Autodesk Fusion 360 part; units mm, degrees
(part 2 of 4)
  spline S104 degree 3 poles (141.5126, -71.1186) (141.7888, -71.118) (142.0126, -70.8942) (142.0127, -70.6185) knots 0 0 0 0 1 1 1 1
  line L150 (142.0127, -70.6185) -> (142.0127, -57.6177)
  spline S105 degree 3 poles (142.0127, -57.6177) (142.0126, -57.342) (141.7888, -57.1181) (141.5126, -57.1177) knots 0 0 0 0 1 1 1 1
  line L151 (141.5126, -57.1177) -> (137.5127, -57.1172)
  line L152 (137.5127, -57.1172) -> (137.5127, -56.6175)
  spline S106 degree 3 poles (137.5127, -56.6175) (137.5126, -56.3418) (137.2888, -56.118) (137.0126, -56.1175) knots 0 0 0 0 1 1 1 1
  line L153 (137.0126, -56.1175) -> (133.0126, -56.1175)
  spline S107 degree 3 poles (133.0126, -56.1175) (132.7365, -56.118) (132.5126, -56.3418) (132.5126, -56.6175) knots 0 0 0 0 1 1 1 1
  line L154 (132.5126, -56.6175) -> (132.5126, -57.1172)
  line L155 (132.5126, -57.1172) -> (128.5126, -57.1177)
  spline S108 degree 3 poles (128.5126, -57.1177) (128.2365, -57.118) (128.0126, -57.342) (128.0126, -57.6177) knots 0 0 0 0 1 1 1 1
  line L156 (128.0126, -57.6177) -> (128.0126, -70.6185)
  spline S109 degree 3 poles (128.0126, -70.6185) (128.0126, -70.8942) (128.2365, -71.1181) (128.5126, -71.1186) knots 0 0 0 0 1 1 1 1
  line L157 (128.5126, -71.1186) -> (132.5126, -71.1191)
  line L158 (132.5126, -71.1191) -> (132.5126, -71.6187)
  spline S110 degree 3 poles (132.5126, -71.6187) (132.5126, -71.8943) (132.7365, -72.1181) (133.0126, -72.1187) knots 0 0 0 0 1 1 1 1
  line L159 (133.0126, -72.1187) -> (137.0126, -72.1187)
  spline S111 degree 3 poles (137.0126, -72.1187) (137.2888, -72.1182) (137.5126, -71.8943) (137.5127, -71.6187) knots 0 0 0 0 1 1 1 1
  spline S112 degree 3 poles (17.9501, -64.9749) (18.2263, -64.9744) (18.4501, -64.7505) (18.4501, -64.4749) knots 0 0 0 0 1 1 1 1
  line L160 (18.4501, -64.4749) -> (18.4501, -63.9754)
  line L161 (18.4501, -63.9754) -> (22.4501, -63.9748)
  spline S113 degree 3 poles (22.4501, -63.9748) (22.7263, -63.9743) (22.9501, -63.7505) (22.9501, -63.4748) knots 0 0 0 0 1 1 1 1
  line L162 (22.9501, -63.4748) -> (22.9501, -50.474)
  spline S114 degree 3 poles (22.9501, -50.474) (22.9501, -50.1982) (22.7263, -49.9743) (22.4501, -49.9739) knots 0 0 0 0 1 1 1 1
  line L163 (22.4501, -49.9739) -> (18.4501, -49.9736)
  line L164 (18.4501, -49.9736) -> (18.4501, -49.474)
  spline S115 degree 3 poles (18.4501, -49.474) (18.4501, -49.1983) (18.2263, -48.9744) (17.9501, -48.9739) knots 0 0 0 0 1 1 1 1
  line L165 (17.9501, -48.9739) -> (13.9501, -48.9739)
  spline S116 degree 3 poles (13.9501, -48.9739) (13.674, -48.9745) (13.4501, -49.1983) (13.4501, -49.474) knots 0 0 0 0 1 1 1 1
  line L166 (13.4501, -49.474) -> (13.4501, -49.9736)
  line L167 (13.4501, -49.9736) -> (9.4501, -49.9739)
  spline S117 degree 3 poles (9.4501, -49.9739) (9.174, -49.9741) (8.9501, -50.1981) (8.9501, -50.4739) knots 0 0 0 0 1 1 1 1
  line L168 (8.9501, -50.4739) -> (8.9501, -63.4747)
  spline S118 degree 3 poles (8.9501, -63.4747) (8.9501, -63.7504) (9.174, -63.9743) (9.4501, -63.9747) knots 0 0 0 0 1 1 1 1
  line L169 (9.4501, -63.9747) -> (13.4501, -63.9753)
  line L170 (13.4501, -63.9753) -> (13.4501, -64.4748)
  spline S119 degree 3 poles (13.4501, -64.4748) (13.4501, -64.7505) (13.674, -64.9743) (13.9501, -64.9749) knots 0 0 0 0 1 1 1 1
  line L171 (13.9501, -64.9749) -> (17.9501, -64.9749)
  line L172 (42.2626, -64.4749) -> (42.2627, -63.9754)
  line L173 (42.2627, -63.9754) -> (46.2626, -63.9748)
  spline S120 degree 3 poles (46.2626, -63.9748) (46.5388, -63.9743) (46.7626, -63.7505) (46.7627, -63.4748) knots 0 0 0 0 1 1 1 1
  line L174 (46.7627, -63.4748) -> (46.7627, -50.474)
  spline S121 degree 3 poles (46.7627, -50.474) (46.7626, -50.1982) (46.5388, -49.9743) (46.2626, -49.9739) knots 0 0 0 0 1 1 1 1
  line L175 (46.2626, -49.9739) -> (42.2627, -49.9734)
  line L176 (42.2627, -49.9734) -> (42.2626, -49.4738)
  spline S122 degree 3 poles (42.2626, -49.4738) (42.2626, -49.1981) (42.0388, -48.9742) (41.7626, -48.9738) knots 0 0 0 0 1 1 1 1
  line L177 (41.7626, -48.9738) -> (37.7626, -48.9738)
  spline S123 degree 3 poles (37.7626, -48.9738) (37.4865, -48.9743) (37.2626, -49.1981) (37.2626, -49.4738) knots 0 0 0 0 1 1 1 1
  line L178 (37.2626, -49.4738) -> (37.2626, -49.9734)
  line L179 (37.2626, -49.9734) -> (33.2626, -49.9739)
  spline S124 degree 3 poles (33.2626, -49.9739) (32.9865, -49.9742) (32.7626, -50.1982) (32.7626, -50.474) knots 0 0 0 0 1 1 1 1
  line L180 (32.7626, -50.474) -> (32.7626, -63.4748)
  spline S125 degree 3 poles (32.7626, -63.4748) (32.7626, -63.7505) (32.9865, -63.9743) (33.2626, -63.9748) knots 0 0 0 0 1 1 1 1
  line L181 (33.2626, -63.9748) -> (37.2626, -63.9754)
  line L182 (37.2626, -63.9754) -> (37.2626, -64.4749)
  spline S126 degree 3 poles (37.2626, -64.4749) (37.2626, -64.7505) (37.4865, -64.9744) (37.7626, -64.9749) knots 0 0 0 0 1 1 1 1
  line L183 (37.7626, -64.9749) -> (41.7626, -64.9749)
  spline S127 degree 3 poles (41.7626, -64.9749) (42.0388, -64.9744) (42.2626, -64.7505) (42.2626, -64.4749) knots 0 0 0 0 1 1 1 1
  line L184 (61.3126, -59.7124) -> (61.3127, -59.2129)
  line L185 (61.3127, -59.2129) -> (65.3126, -59.2123)
  spline S128 degree 3 poles (65.3126, -59.2123) (65.5888, -59.2118) (65.8126, -58.988) (65.8127, -58.7123) knots 0 0 0 0 1 1 1 1
  line L186 (65.8127, -58.7123) -> (65.8127, -45.7115)
  spline S129 degree 3 poles (65.8127, -45.7115) (65.8126, -45.4357) (65.5888, -45.2118) (65.3126, -45.2114) knots 0 0 0 0 1 1 1 1
  line L187 (65.3126, -45.2114) -> (61.3127, -45.2109)
  line L188 (61.3127, -45.2109) -> (61.3126, -44.7113)
  spline S130 degree 3 poles (61.3126, -44.7113) (61.3126, -44.4356) (61.0888, -44.2117) (60.8126, -44.2113) knots 0 0 0 0 1 1 1 1
  line L189 (60.8126, -44.2113) -> (56.8126, -44.2113)
  spline S131 degree 3 poles (56.8126, -44.2113) (56.5365, -44.2118) (56.3126, -44.4356) (56.3126, -44.7113) knots 0 0 0 0 1 1 1 1
  line L190 (56.3126, -44.7113) -> (56.3126, -45.2109)
  line L191 (56.3126, -45.2109) -> (52.3126, -45.2114)
  spline S132 degree 3 poles (52.3126, -45.2114) (52.0365, -45.2117) (51.8126, -45.4357) (51.8126, -45.7115) knots 0 0 0 0 1 1 1 1
  line L192 (51.8126, -45.7115) -> (51.8126, -58.7123)
  spline S133 degree 3 poles (51.8126, -58.7123) (51.8126, -58.988) (52.0365, -59.2118) (52.3126, -59.2123) knots 0 0 0 0 1 1 1 1
  line L193 (52.3126, -59.2123) -> (56.3126, -59.2129)
  line L194 (56.3126, -59.2129) -> (56.3126, -59.7124)
  spline S134 degree 3 poles (56.3126, -59.7124) (56.3126, -59.988) (56.5365, -60.2119) (56.8126, -60.2124) knots 0 0 0 0 1 1 1 1
  line L195 (56.8126, -60.2124) -> (60.8126, -60.2124)
  spline S135 degree 3 poles (60.8126, -60.2124) (61.0888, -60.2119) (61.3126, -59.988) (61.3126, -59.7124) knots 0 0 0 0 1 1 1 1
  line L196 (80.3626, -57.3312) -> (80.3627, -56.8316)
  line L197 (80.3627, -56.8316) -> (84.3626, -56.8311)
  spline S136 degree 3 poles (84.3626, -56.8311) (84.6388, -56.8305) (84.8626, -56.6067) (84.8627, -56.331) knots 0 0 0 0 1 1 1 1
  line L198 (84.8627, -56.331) -> (84.8627, -43.3302)
  spline S137 degree 3 poles (84.8627, -43.3302) (84.8626, -43.0545) (84.6388, -42.8306) (84.3626, -42.8302) knots 0 0 0 0 1 1 1 1
  line L199 (84.3626, -42.8302) -> (80.3627, -42.8297)
  line L200 (80.3627, -42.8297) -> (80.3626, -42.33)
  spline S138 degree 3 poles (80.3626, -42.33) (80.3626, -42.0543) (80.1388, -41.8305) (79.8626, -41.83) knots 0 0 0 0 1 1 1 1
  line L201 (79.8626, -41.83) -> (75.8626, -41.83)
  spline S139 degree 3 poles (75.8626, -41.83) (75.5865, -41.8305) (75.3626, -42.0543) (75.3626, -42.33) knots 0 0 0 0 1 1 1 1
  line L202 (75.3626, -42.33) -> (75.3626, -42.8297)
  line L203 (75.3626, -42.8297) -> (71.3626, -42.8302)
  spline S140 degree 3 poles (71.3626, -42.8302) (71.0865, -42.8305) (70.8626, -43.0545) (70.8626, -43.3302) knots 0 0 0 0 1 1 1 1
  line L204 (70.8626, -43.3302) -> (70.8626, -56.331)
  spline S141 degree 3 poles (70.8626, -56.331) (70.8626, -56.6067) (71.0865, -56.8306) (71.3626, -56.8311) knots 0 0 0 0 1 1 1 1
  line L205 (71.3626, -56.8311) -> (75.3626, -56.8316)
  line L206 (75.3626, -56.8316) -> (75.3626, -57.3312)
  spline S142 degree 3 poles (75.3626, -57.3312) (75.3626, -57.6068) (75.5865, -57.8306) (75.8626, -57.8312) knots 0 0 0 0 1 1 1 1
  line L207 (75.8626, -57.8312) -> (79.8626, -57.8312)
  spline S143 degree 3 poles (79.8626, -57.8312) (80.1388, -57.8307) (80.3626, -57.6068) (80.3626, -57.3312) knots 0 0 0 0 1 1 1 1
  line L208 (99.4126, -59.7124) -> (99.4127, -59.2129)
  line L209 (99.4127, -59.2129) -> (103.4126, -59.2123)
  spline S144 degree 3 poles (103.4126, -59.2123) (103.6888, -59.2118) (103.9126, -58.988) (103.9127, -58.7123) knots 0 0 0 0 1 1 1 1
  line L210 (103.9127, -58.7123) -> (103.9127, -45.7115)
  spline S145 degree 3 poles (103.9127, -45.7115) (103.9126, -45.4357) (103.6888, -45.2118) (103.4126, -45.2114) knots 0 0 0 0 1 1 1 1
  line L211 (103.4126, -45.2114) -> (99.4127, -45.2109)
  line L212 (99.4127, -45.2109) -> (99.4126, -44.7113)
  spline S146 degree 3 poles (99.4126, -44.7113) (99.4126, -44.4356) (99.1888, -44.2117) (98.9126, -44.2113) knots 0 0 0 0 1 1 1 1
  line L213 (98.9126, -44.2113) -> (94.9126, -44.2113)
  spline S147 degree 3 poles (94.9126, -44.2113) (94.6365, -44.2118) (94.4126, -44.4356) (94.4126, -44.7113) knots 0 0 0 0 1 1 1 1
  line L214 (94.4126, -44.7113) -> (94.4126, -45.2109)
  line L215 (94.4126, -45.2109) -> (90.4126, -45.2114)
  spline S148 degree 3 poles (90.4126, -45.2114) (90.1365, -45.2117) (89.9126, -45.4357) (89.9126, -45.7115) knots 0 0 0 0 1 1 1 1
  line L216 (89.9126, -45.7115) -> (89.9126, -58.7123)
  spline S149 degree 3 poles (89.9126, -58.7123) (89.9126, -58.988) (90.1365, -59.2118) (90.4126, -59.2123) knots 0 0 0 0 1 1 1 1
  line L217 (90.4126, -59.2123) -> (94.4126, -59.2129)
  line L218 (94.4126, -59.2129) -> (94.4126, -59.7124)
  spline S150 degree 3 poles (94.4126, -59.7124) (94.4126, -59.988) (94.6365, -60.2119) (94.9126, -60.2124) knots 0 0 0 0 1 1 1 1
  line L219 (94.9126, -60.2124) -> (98.9126, -60.2124)
  spline S151 degree 3 poles (98.9126, -60.2124) (99.1888, -60.2119) (99.4126, -59.988) (99.4126, -59.7124) knots 0 0 0 0 1 1 1 1
  line L220 (118.4626, -62.0937) -> (118.4627, -61.5941)
  line L221 (118.4627, -61.5941) -> (122.4626, -61.5936)
  spline S152 degree 3 poles (122.4626, -61.5936) (122.7388, -61.593) (122.9626, -61.3692) (122.9627, -61.0935) knots 0 0 0 0 1 1 1 1
  line L222 (122.9627, -61.0935) -> (122.9627, -48.0927)
  spline S153 degree 3 poles (122.9627, -48.0927) (122.9626, -47.817) (122.7388, -47.5931) (122.4626, -47.5927) knots 0 0 0 0 1 1 1 1
  line L223 (122.4626, -47.5927) -> (118.4627, -47.5922)
  line L224 (118.4627, -47.5922) -> (118.4626, -47.0925)
  spline S154 degree 3 poles (118.4626, -47.0925) (118.4626, -46.8168) (118.2388, -46.593) (117.9626, -46.5925) knots 0 0 0 0 1 1 1 1
  line L225 (117.9626, -46.5925) -> (113.9626, -46.5925)
  spline S155 degree 3 poles (113.9626, -46.5925) (113.6865, -46.593) (113.4626, -46.8168) (113.4626, -47.0925) knots 0 0 0 0 1 1 1 1
  line L226 (113.4626, -47.0925) -> (113.4626, -47.5922)
  line L227 (113.4626, -47.5922) -> (109.4626, -47.5927)
  spline S156 degree 3 poles (109.4626, -47.5927) (109.1865, -47.593) (108.9626, -47.817) (108.9626, -48.0927) knots 0 0 0 0 1 1 1 1
  line L228 (108.9626, -48.0927) -> (108.9626, -61.0935)
  spline S157 degree 3 poles (108.9626, -61.0935) (108.9626, -61.3692) (109.1865, -61.5931) (109.4626, -61.5936) knots 0 0 0 0 1 1 1 1
  line L229 (109.4626, -61.5936) -> (113.4626, -61.5941)
  line L230 (113.4626, -61.5941) -> (113.4626, -62.0937)
  spline S158 degree 3 poles (113.4626, -62.0937) (113.4626, -62.3693) (113.6865, -62.5931) (113.9626, -62.5937) knots 0 0 0 0 1 1 1 1
  line L231 (113.9626, -62.5937) -> (117.9626, -62.5937)
  spline S159 degree 3 poles (117.9626, -62.5937) (118.2388, -62.5932) (118.4626, -62.3693) (118.4626, -62.0937) knots 0 0 0 0 1 1 1 1
  spline S160 degree 3 poles (17.9501, -45.9249) (18.2263, -45.9244) (18.4501, -45.7005) (18.4501, -45.4249) knots 0 0 0 0 1 1 1 1
  line L232 (18.4501, -45.4249) -> (18.4501, -44.9254)
  line L233 (18.4501, -44.9254) -> (22.4501, -44.9248)
  spline S161 degree 3 poles (22.4501, -44.9248) (22.7263, -44.9243) (22.9501, -44.7005) (22.9501, -44.4248) knots 0 0 0 0 1 1 1 1
  line L234 (22.9501, -44.4248) -> (22.9501, -31.424)
  spline S162 degree 3 poles (22.9501, -31.424) (22.9501, -31.1482) (22.7263, -30.9243) (22.4501, -30.9239) knots 0 0 0 0 1 1 1 1
  line L235 (22.4501, -30.9239) -> (18.4501, -30.9236)
  line L236 (18.4501, -30.9236) -> (18.4501, -30.424)
  spline S163 degree 3 poles (18.4501, -30.424) (18.4501, -30.1483) (18.2263, -29.9244) (17.9501, -29.9239) knots 0 0 0 0 1 1 1 1
  line L237 (17.9501, -29.9239) -> (13.9501, -29.9239)
  spline S164 degree 3 poles (13.9501, -29.9239) (13.674, -29.9245) (13.4501, -30.1483) (13.4501, -30.424) knots 0 0 0 0 1 1 1 1
  line L238 (13.4501, -30.424) -> (13.4501, -30.9236)
  line L239 (13.4501, -30.9236) -> (9.4501, -30.9239)
  spline S165 degree 3 poles (9.4501, -30.9239) (9.174, -30.9244) (8.9501, -31.1481) (8.9501, -31.4239) knots 0 0 0 0 1 1 1 1
  line L240 (8.9501, -31.4239) -> (8.9501, -44.4247)
  spline S166 degree 3 poles (8.9501, -44.4247) (8.9501, -44.7004) (9.174, -44.9243) (9.4501, -44.9247) knots 0 0 0 0 1 1 1 1
  line L241 (9.4501, -44.9247) -> (13.4501, -44.9253)
  line L242 (13.4501, -44.9253) -> (13.4501, -45.4248)
  spline S167 degree 3 poles (13.4501, -45.4248) (13.4501, -45.7005) (13.674, -45.9243) (13.9501, -45.9249) knots 0 0 0 0 1 1 1 1
  line L243 (13.9501, -45.9249) -> (17.9501, -45.9249)
  line L244 (42.2626, -45.4249) -> (42.2627, -44.9254)
  line L245 (42.2627, -44.9254) -> (46.2626, -44.9248)
  spline S168 degree 3 poles (46.2626, -44.9248) (46.5388, -44.9243) (46.7626, -44.7005) (46.7627, -44.4248) knots 0 0 0 0 1 1 1 1
  line L246 (46.7627, -44.4248) -> (46.7627, -31.424)
  spline S169 degree 3 poles (46.7627, -31.424) (46.7626, -31.1482) (46.5388, -30.9243) (46.2626, -30.9239) knots 0 0 0 0 1 1 1 1
  line L247 (46.2626, -30.9239) -> (42.2627, -30.9237)
  line L248 (42.2627, -30.9237) -> (42.2626, -30.424)
  spline S170 degree 3 poles (42.2626, -30.424) (42.2626, -30.1483) (42.0388, -29.9245) (41.7626, -29.924) knots 0 0 0 0 1 1 1 1
  line L249 (41.7626, -29.924) -> (37.7626, -29.924)
  spline S171 degree 3 poles (37.7626, -29.924) (37.4865, -29.9245) (37.2626, -30.1483) (37.2626, -30.424) knots 0 0 0 0 1 1 1 1
  line L250 (37.2626, -30.424) -> (37.2626, -30.9237)
  line L251 (37.2626, -30.9237) -> (33.2626, -30.9239)
  spline S172 degree 3 poles (33.2626, -30.9239) (32.9865, -30.9245) (32.7626, -31.1482) (32.7626, -31.424) knots 0 0 0 0 1 1 1 1
  line L252 (32.7626, -31.424) -> (32.7626, -44.4248)
  spline S173 degree 3 poles (32.7626, -44.4248) (32.7626, -44.7005) (32.9865, -44.9243) (33.2626, -44.9248) knots 0 0 0 0 1 1 1 1
  line L253 (33.2626, -44.9248) -> (37.2626, -44.9254)
  line L254 (37.2626, -44.9254) -> (37.2626, -45.4249)
  spline S174 degree 3 poles (37.2626, -45.4249) (37.2626, -45.7005) (37.4865, -45.9244) (37.7626, -45.9249) knots 0 0 0 0 1 1 1 1
  line L255 (37.7626, -45.9249) -> (41.7626, -45.9249)
  spline S175 degree 3 poles (41.7626, -45.9249) (42.0388, -45.9244) (42.2626, -45.7005) (42.2626, -45.4249) knots 0 0 0 0 1 1 1 1
  line L256 (61.3126, -40.6624) -> (61.3127, -40.1629)
  line L257 (61.3127, -40.1629) -> (65.3126, -40.1623)
  spline S176 degree 3 poles (65.3126, -40.1623) (65.5888, -40.1618) (65.8126, -39.938) (65.8127, -39.6623) knots 0 0 0 0 1 1 1 1
  line L258 (65.8127, -39.6623) -> (65.8127, -26.6615)
  spline S177 degree 3 poles (65.8127, -26.6615) (65.8126, -26.3858) (65.5888, -26.1619) (65.3126, -26.1615) knots 0 0 0 0 1 1 1 1
  line L259 (65.3126, -26.1615) -> (61.3127, -26.1611)
  line L260 (61.3127, -26.1611) -> (61.3126, -25.6615)
  spline S178 degree 3 poles (61.3126, -25.6615) (61.3126, -25.3858) (61.0888, -25.1619) (60.8126, -25.1614) knots 0 0 0 0 1 1 1 1
  line L261 (60.8126, -25.1614) -> (56.8126, -25.1614)
  spline S179 degree 3 poles (56.8126, -25.1614) (56.5365, -25.1619) (56.3126, -25.3858) (56.3126, -25.6615) knots 0 0 0 0 1 1 1 1
  line L262 (56.3126, -25.6615) -> (56.3126, -26.1611)
  line L263 (56.3126, -26.1611) -> (52.3126, -26.1615)
  spline S180 degree 3 poles (52.3126, -26.1615) (52.0365, -26.1619) (51.8126, -26.3858) (51.8126, -26.6615) knots 0 0 0 0 1 1 1 1
  line L264 (51.8126, -26.6615) -> (51.8126, -39.6623)
  spline S181 degree 3 poles (51.8126, -39.6623) (51.8126, -39.938) (52.0365, -40.1619) (52.3126, -40.1624) knots 0 0 0 0 1 1 1 1
  line L265 (52.3126, -40.1624) -> (56.3126, -40.1629)
  line L266 (56.3126, -40.1629) -> (56.3126, -40.6625)
  spline S182 degree 3 poles (56.3126, -40.6625) (56.3126, -40.9381) (56.5365, -41.1619) (56.8126, -41.1625) knots 0 0 0 0 1 1 1 1
  line L267 (56.8126, -41.1625) -> (60.8126, -41.1625)
  spline S183 degree 3 poles (60.8126, -41.1625) (61.0888, -41.162) (61.3126, -40.9381) (61.3126, -40.6624) knots 0 0 0 0 1 1 1 1
  line L268 (80.3626, -38.2812) -> (80.3627, -37.7816)
  line L269 (80.3627, -37.7816) -> (84.3626, -37.7811)
  spline S184 degree 3 poles (84.3626, -37.7811) (84.6388, -37.7805) (84.8626, -37.5567) (84.8627, -37.281) knots 0 0 0 0 1 1 1 1
  line L270 (84.8627, -37.281) -> (84.8627, -24.2803)
  spline S185 degree 3 poles (84.8627, -24.2803) (84.8626, -24.0045) (84.6388, -23.7806) (84.3626, -23.7803) knots 0 0 0 0 1 1 1 1
  line L271 (84.3626, -23.7803) -> (80.3627, -23.7799)
  line L272 (80.3627, -23.7799) -> (80.3626, -23.2802)
  spline S186 degree 3 poles (80.3626, -23.2802) (80.3626, -23.0045) (80.1388, -22.7806) (79.8626, -22.7802) knots 0 0 0 0 1 1 1 1
  line L273 (79.8626, -22.7802) -> (75.8626, -22.7802)
  spline S187 degree 3 poles (75.8626, -22.7802) (75.5865, -22.7806) (75.3626, -23.0045) (75.3626, -23.2802) knots 0 0 0 0 1 1 1 1
  line L274 (75.3626, -23.2802) -> (75.3626, -23.7799)
  line L275 (75.3626, -23.7799) -> (71.3626, -23.7803)
  spline S188 degree 3 poles (71.3626, -23.7803) (71.0865, -23.7806) (70.8626, -24.0045) (70.8626, -24.2803) knots 0 0 0 0 1 1 1 1
  line L276 (70.8626, -24.2803) -> (70.8626, -37.2811)
  spline S189 degree 3 poles (70.8626, -37.2811) (70.8626, -37.5568) (71.0865, -37.7806) (71.3626, -37.7811) knots 0 0 0 0 1 1 1 1
  line L277 (71.3626, -37.7811) -> (75.3626, -37.7817)
  line L278 (75.3626, -37.7817) -> (75.3626, -38.2812)
  spline S190 degree 3 poles (75.3626, -38.2812) (75.3626, -38.5568) (75.5865, -38.7807) (75.8626, -38.7812) knots 0 0 0 0 1 1 1 1
  line L279 (75.8626, -38.7812) -> (79.8626, -38.7812)
  spline S191 degree 3 poles (79.8626, -38.7812) (80.1388, -38.7807) (80.3626, -38.5568) (80.3626, -38.2812) knots 0 0 0 0 1 1 1 1
  line L280 (99.4126, -40.6624) -> (99.4127, -40.1629)
  line L281 (99.4127, -40.1629) -> (103.4126, -40.1623)
  spline S192 degree 3 poles (103.4126, -40.1623) (103.6888, -40.1618) (103.9126, -39.938) (103.9127, -39.6623) knots 0 0 0 0 1 1 1 1
  line L282 (103.9127, -39.6623) -> (103.9127, -26.6615)
  spline S193 degree 3 poles (103.9127, -26.6615) (103.9126, -26.3858) (103.6888, -26.1619) (103.4126, -26.1615) knots 0 0 0 0 1 1 1 1
  line L283 (103.4126, -26.1615) -> (99.4127, -26.1611)
  line L284 (99.4127, -26.1611) -> (99.4126, -25.6615)
  spline S194 degree 3 poles (99.4126, -25.6615) (99.4126, -25.3858) (99.1888, -25.1619) (98.9126, -25.1614) knots 0 0 0 0 1 1 1 1
  line L285 (98.9126, -25.1614) -> (94.9126, -25.1614)
  spline S195 degree 3 poles (94.9126, -25.1614) (94.6365, -25.1619) (94.4126, -25.3858) (94.4126, -25.6615) knots 0 0 0 0 1 1 1 1
  line L286 (94.4126, -25.6615) -> (94.4126, -26.1611)
  line L287 (94.4126, -26.1611) -> (90.4126, -26.1615)
  spline S196 degree 3 poles (90.4126, -26.1615) (90.1365, -26.1619) (89.9126, -26.3858) (89.9126, -26.6615) knots 0 0 0 0 1 1 1 1
  line L288 (89.9126, -26.6615) -> (89.9126, -39.6623)
  spline S197 degree 3 poles (89.9126, -39.6623) (89.9126, -39.938) (90.1365, -40.1619) (90.4126, -40.1624) knots 0 0 0 0 1 1 1 1
  line L289 (90.4126, -40.1624) -> (94.4126, -40.1629)
  line L290 (94.4126, -40.1629) -> (94.4126, -40.6625)
  spline S198 degree 3 poles (94.4126, -40.6625) (94.4126, -40.9381) (94.6365, -41.1619) (94.9126, -41.1625) knots 0 0 0 0 1 1 1 1
  line L291 (94.9126, -41.1625) -> (98.9126, -41.1625)
  spline S199 degree 3 poles (98.9126, -41.1625) (99.1888, -41.162) (99.4126, -40.9381) (99.4126, -40.6624) knots 0 0 0 0 1 1 1 1
  line L292 (118.4626, -43.0437) -> (118.4627, -42.5441)
  line L293 (118.4627, -42.5441) -> (122.4626, -42.5436)
  spline S200 degree 3 poles (122.4626, -42.5436) (122.7388, -42.543) (122.9626, -42.3192) (122.9627, -42.0435) knots 0 0 0 0 1 1 1 1
  line L294 (122.9627, -42.0435) -> (122.9627, -29.0427)
  spline S201 degree 3 poles (122.9627, -29.0427) (122.9626, -28.7669) (122.7388, -28.5431) (122.4626, -28.5427) knots 0 0 0 0 1 1 1 1
  line L295 (122.4626, -28.5427) -> (118.4627, -28.5424)
  line L296 (118.4627, -28.5424) -> (118.4626, -28.0428)
  spline S202 degree 3 poles (118.4626, -28.0428) (118.4626, -27.7671) (118.2388, -27.5432) (117.9626, -27.5428) knots 0 0 0 0 1 1 1 1
  line L297 (117.9626, -27.5428) -> (113.9626, -27.5428)
  spline S203 degree 3 poles (113.9626, -27.5428) (113.6865, -27.5432) (113.4626, -27.7671) (113.4626, -28.0428) knots 0 0 0 0 1 1 1 1
  line L298 (113.4626, -28.0428) -> (113.4626, -28.5424)
  line L299 (113.4626, -28.5424) -> (109.4626, -28.5427)
  spline S204 degree 3 poles (109.4626, -28.5427) (109.1865, -28.5432) (108.9626, -28.767) (108.9626, -29.0427) knots 0 0 0 0 1 1 1 1
  line L300 (108.9626, -29.0427) -> (108.9626, -42.0435)
  spline S205 degree 3 poles (108.9626, -42.0435) (108.9626, -42.3192) (109.1865, -42.5431) (109.4626, -42.5436) knots 0 0 0 0 1 1 1 1
  line L301 (109.4626, -42.5436) -> (113.4626, -42.5441)
  line L302 (113.4626, -42.5441) -> (113.4626, -43.0437)
  spline S206 degree 3 poles (113.4626, -43.0437) (113.4626, -43.3193) (113.6865, -43.5431) (113.9626, -43.5437) knots 0 0 0 0 1 1 1 1
  line L303 (113.9626, -43.5437) -> (117.9626, -43.5437)
  spline S207 degree 3 poles (117.9626, -43.5437) (118.2388, -43.5432) (118.4626, -43.3193) (118.4626, -43.0437) knots 0 0 0 0 1 1 1 1
  spline S208 degree 3 poles (17.9501, -26.8749) (18.2263, -26.8744) (18.4501, -26.6505) (18.4501, -26.3749) knots 0 0 0 0 1 1 1 1
  line L304 (18.4501, -26.3749) -> (18.4501, -25.8754)
  line L305 (18.4501, -25.8754) -> (22.4501, -25.8749)
  spline S209 degree 3 poles (22.4501, -25.8749) (22.7263, -25.8744) (22.9501, -25.6505) (22.9501, -25.3748) knots 0 0 0 0 1 1 1 1
  line L306 (22.9501, -25.3748) -> (22.9501, -12.374)
  spline S210 degree 3 poles (22.9501, -12.374) (22.9501, -12.0983) (22.7263, -11.8744) (22.4501, -11.874) knots 0 0 0 0 1 1 1 1
  line L307 (22.4501, -11.874) -> (18.4501, -11.8736)
  line L308 (18.4501, -11.8736) -> (18.4501, -11.374)
  spline S211 degree 3 poles (18.4501, -11.374) (18.4501, -11.0983) (18.2263, -10.8744) (17.9501, -10.8739) knots 0 0 0 0 1 1 1 1
  line L309 (17.9501, -10.8739) -> (13.9501, -10.8739)
  spline S212 degree 3 poles (13.9501, -10.8739) (13.674, -10.8744) (13.4501, -11.0983) (13.4501, -11.374) knots 0 0 0 0 1 1 1 1
  line L310 (13.4501, -11.374) -> (13.4501, -11.8736)
  line L311 (13.4501, -11.8736) -> (9.4501, -11.874)
  spline S213 degree 3 poles (9.4501, -11.874) (9.174, -11.8744) (8.9501, -12.0983) (8.9501, -12.374) knots 0 0 0 0 1 1 1 1
  line L312 (8.9501, -12.374) -> (8.9501, -25.3748)
  spline S214 degree 3 poles (8.9501, -25.3748) (8.9501, -25.6505) (9.174, -25.8744) (9.4501, -25.8749) knots 0 0 0 0 1 1 1 1
  line L313 (9.4501, -25.8749) -> (13.4501, -25.8754)
  line L314 (13.4501, -25.8754) -> (13.4501, -26.3749)
  spline S215 degree 3 poles (13.4501, -26.3749) (13.4501, -26.6505) (13.674, -26.8744) (13.9501, -26.8749) knots 0 0 0 0 1 1 1 1
  line L315 (13.9501, -26.8749) -> (17.9501, -26.8749)
  line L316 (42.2626, -26.3749) -> (42.2627, -25.8754)
  line L317 (42.2627, -25.8754) -> (46.2626, -25.8749)
  spline S216 degree 3 poles (46.2626, -25.8749) (46.5388, -25.8744) (46.7626, -25.6505) (46.7627, -25.3748) knots 0 0 0 0 1 1 1 1
  line L318 (46.7627, -25.3748) -> (46.7627, -12.374)
  spline S217 degree 3 poles (46.7627, -12.374) (46.7626, -12.0983) (46.5388, -11.8744) (46.2626, -11.874) knots 0 0 0 0 1 1 1 1
  line L319 (46.2626, -11.874) -> (42.2627, -11.8736)
  line L320 (42.2627, -11.8736) -> (42.2626, -11.374)
  spline S218 degree 3 poles (42.2626, -11.374) (42.2626, -11.0983) (42.0388, -10.8744) (41.7626, -10.8739) knots 0 0 0 0 1 1 1 1
  line L321 (41.7626, -10.8739) -> (37.7626, -10.8739)
  spline S219 degree 3 poles (37.7626, -10.8739) (37.4865, -10.8744) (37.2626, -11.0983) (37.2626, -11.374) knots 0 0 0 0 1 1 1 1
  line L322 (37.2626, -11.374) -> (37.2626, -11.8736)
  line L323 (37.2626, -11.8736) -> (33.2626, -11.874)
  spline S220 degree 3 poles (33.2626, -11.874) (32.9865, -11.8744) (32.7626, -12.0983) (32.7626, -12.374) knots 0 0 0 0 1 1 1 1
  line L324 (32.7626, -12.374) -> (32.7626, -25.3748)
  spline S221 degree 3 poles (32.7626, -25.3748) (32.7626, -25.6505) (32.9865, -25.8744) (33.2626, -25.8749) knots 0 0 0 0 1 1 1 1
  line L325 (33.2626, -25.8749) -> (37.2626, -25.8754)
  line L326 (37.2626, -25.8754) -> (37.2626, -26.3749)
  spline S222 degree 3 poles (37.2626, -26.3749) (37.2626, -26.6505) (37.4865, -26.8744) (37.7626, -26.8749) knots 0 0 0 0 1 1 1 1
  line L327 (37.7626, -26.8749) -> (41.7626, -26.8749)
  spline S223 degree 3 poles (41.7626, -26.8749) (42.0388, -26.8744) (42.2626, -26.6505) (42.2626, -26.3749) knots 0 0 0 0 1 1 1 1
  line L328 (61.3126, -21.6124) -> (61.3127, -21.1129)
  line L329 (61.3127, -21.1129) -> (65.3126, -21.1124)
  spline S224 degree 3 poles (65.3126, -21.1124) (65.5888, -21.1119) (65.8126, -20.888) (65.8127, -20.6123) knots 0 0 0 0 1 1 1 1
  line L330 (65.8127, -20.6123) -> (65.8127, -7.6115)
  spline S225 degree 3 poles (65.8127, -7.6115) (65.8126, -7.3358) (65.5888, -7.1119) (65.3126, -7.1115) knots 0 0 0 0 1 1 1 1
  line L331 (65.3126, -7.1115) -> (61.3127, -7.1111)
  line L332 (61.3127, -7.1111) -> (61.3126, -6.6115)
  spline S226 degree 3 poles (61.3126, -6.6115) (61.3126, -6.3358) (61.0888, -6.1119) (60.8126, -6.1114) knots 0 0 0 0 1 1 1 1
  line L333 (60.8126, -6.1114) -> (56.8126, -6.1114)
  spline S227 degree 3 poles (56.8126, -6.1114) (56.5365, -6.1119) (56.3126, -6.3358) (56.3126, -6.6115) knots 0 0 0 0 1 1 1 1
  line L334 (56.3126, -6.6115) -> (56.3126, -7.1111)
  line L335 (56.3126, -7.1111) -> (52.3126, -7.1115)
  spline S228 degree 3 poles (52.3126, -7.1115) (52.0365, -7.1119) (51.8126, -7.3358) (51.8126, -7.6115) knots 0 0 0 0 1 1 1 1
  line L336 (51.8126, -7.6115) -> (51.8126, -20.6123)
  spline S229 degree 3 poles (51.8126, -20.6123) (51.8126, -20.888) (52.0365, -21.1119) (52.3126, -21.1124) knots 0 0 0 0 1 1 1 1
  line L337 (52.3126, -21.1124) -> (56.3126, -21.1129)
  line L338 (56.3126, -21.1129) -> (56.3126, -21.6124)
  spline S230 degree 3 poles (56.3126, -21.6124) (56.3126, -21.888) (56.5365, -22.1119) (56.8126, -22.1124) knots 0 0 0 0 1 1 1 1
  line L339 (56.8126, -22.1124) -> (60.8126, -22.1124)
  spline S231 degree 3 poles (60.8126, -22.1124) (61.0888, -22.1119) (61.3126, -21.888) (61.3126, -21.6124) knots 0 0 0 0 1 1 1 1
  line L340 (80.3626, -19.2312) -> (80.3627, -18.7316)
  line L341 (80.3627, -18.7316) -> (84.3626, -18.7311)
  spline S232 degree 3 poles (84.3626, -18.7311) (84.6388, -18.7307) (84.8626, -18.5068) (84.8627, -18.2311) knots 0 0 0 0 1 1 1 1
  line L342 (84.8627, -18.2311) -> (84.8627, -5.2303)
  spline S233 degree 3 poles (84.8627, -5.2303) (84.8626, -4.9545) (84.6388, -4.7306) (84.3626, -4.7303) knots 0 0 0 0 1 1 1 1
  line L343 (84.3626, -4.7303) -> (80.3627, -4.7299)
  line L344 (80.3627, -4.7299) -> (80.3626, -4.2302)
  spline S234 degree 3 poles (80.3626, -4.2302) (80.3626, -3.9545) (80.1388, -3.7306) (79.8626, -3.7302) knots 0 0 0 0 1 1 1 1
  line L345 (79.8626, -3.7302) -> (75.8626, -3.7302)
  spline S235 degree 3 poles (75.8626, -3.7302) (75.5865, -3.7306) (75.3626, -3.9545) (75.3626, -4.2302) knots 0 0 0 0 1 1 1 1
  line L346 (75.3626, -4.2302) -> (75.3626, -4.7299)
  line L347 (75.3626, -4.7299) -> (71.3626, -4.7303)
  spline S236 degree 3 poles (71.3626, -4.7303) (71.0865, -4.7306) (70.8626, -4.9545) (70.8626, -5.2303) knots 0 0 0 0 1 1 1 1
  line L348 (70.8626, -5.2303) -> (70.8626, -18.2311)
  spline S237 degree 3 poles (70.8626, -18.2311) (70.8626, -18.5068) (71.0865, -18.7306) (71.3626, -18.7311) knots 0 0 0 0 1 1 1 1
  line L349 (71.3626, -18.7311) -> (75.3626, -18.7316)
  line L350 (75.3626, -18.7316) -> (75.3626, -19.2312)
  spline S238 degree 3 poles (75.3626, -19.2312) (75.3626, -19.5068) (75.5865, -19.7306) (75.8626, -19.7312) knots 0 0 0 0 1 1 1 1
  line L351 (75.8626, -19.7312) -> (79.8626, -19.7312)
  spline S239 degree 3 poles (79.8626, -19.7312) (80.1388, -19.7306) (80.3626, -19.5068) (80.3626, -19.2312) knots 0 0 0 0 1 1 1 1
  line L352 (99.4126, -21.6124) -> (99.4127, -21.1129)
  line L353 (99.4127, -21.1129) -> (103.4126, -21.1124)
  spline S240 degree 3 poles (103.4126, -21.1124) (103.6888, -21.1119) (103.9126, -20.888) (103.9127, -20.6123) knots 0 0 0 0 1 1 1 1
  line L354 (103.9127, -20.6123) -> (103.9127, -7.6115)
  spline S241 degree 3 poles (103.9127, -7.6115) (103.9126, -7.3358) (103.6888, -7.1119) (103.4126, -7.1115) knots 0 0 0 0 1 1 1 1
  line L355 (103.4126, -7.1115) -> (99.4127, -7.1111)
  line L356 (99.4127, -7.1111) -> (99.4126, -6.6115)
  spline S242 degree 3 poles (99.4126, -6.6115) (99.4126, -6.3358) (99.1888, -6.1119) (98.9126, -6.1114) knots 0 0 0 0 1 1 1 1
  line L357 (98.9126, -6.1114) -> (94.9126, -6.1114)
  spline S243 degree 3 poles (94.9126, -6.1114) (94.6365, -6.1119) (94.4126, -6.3358) (94.4126, -6.6115) knots 0 0 0 0 1 1 1 1
  line L358 (94.4126, -6.6115) -> (94.4126, -7.1111)
  line L359 (94.4126, -7.1111) -> (90.4126, -7.1115)
  spline S244 degree 3 poles (90.4126, -7.1115) (90.1365, -7.1119) (89.9126, -7.3358) (89.9126, -7.6115) knots 0 0 0 0 1 1 1 1
  line L360 (89.9126, -7.6115) -> (89.9126, -20.6123)
  spline S245 degree 3 poles (89.9126, -20.6123) (89.9126, -20.888) (90.1365, -21.1119) (90.4126, -21.1124) knots 0 0 0 0 1 1 1 1
  line L361 (90.4126, -21.1124) -> (94.4126, -21.1129)
  line L362 (94.4126, -21.1129) -> (94.4126, -21.6124)
  spline S246 degree 3 poles (94.4126, -21.6124) (94.4126, -21.888) (94.6365, -22.1119) (94.9126, -22.1124) knots 0 0 0 0 1 1 1 1
  line L363 (94.9126, -22.1124) -> (98.9126, -22.1124)
  spline S247 degree 3 poles (98.9126, -22.1124) (99.1888, -22.1119) (99.4126, -21.888) (99.4126, -21.6124) knots 0 0 0 0 1 1 1 1
  line L364 (118.4626, -23.9937) -> (118.4627, -23.4941)
  line L365 (118.4627, -23.4941) -> (122.4626, -23.4936)
  spline S248 degree 3 poles (122.4626, -23.4936) (122.7388, -23.4932) (122.9626, -23.2693) (122.9627, -22.9936) knots 0 0 0 0 1 1 1 1
  line L366 (122.9627, -22.9936) -> (122.9627, -9.9928)
  spline S249 degree 3 poles (122.9627, -9.9928) (122.9626, -9.717) (122.7388, -9.4931) (122.4626, -9.4928) knots 0 0 0 0 1 1 1 1
  line L367 (122.4626, -9.4928) -> (118.4627, -9.4924)
  line L368 (118.4627, -9.4924) -> (118.4626, -8.9927)
  spline S250 degree 3 poles (118.4626, -8.9927) (118.4626, -8.717) (118.2388, -8.4931) (117.9626, -8.4927) knots 0 0 0 0 1 1 1 1
  line L369 (117.9626, -8.4927) -> (113.9626, -8.4927)
  spline S251 degree 3 poles (113.9626, -8.4927) (113.6865, -8.4931) (113.4626, -8.717) (113.4626, -8.9927) knots 0 0 0 0 1 1 1 1
  line L370 (113.4626, -8.9927) -> (113.4626, -9.4924)
  line L371 (113.4626, -9.4924) -> (109.4626, -9.4928)
  spline S252 degree 3 poles (109.4626, -9.4928) (109.1865, -9.4931) (108.9626, -9.717) (108.9626, -9.9928) knots 0 0 0 0 1 1 1 1
  line L372 (108.9626, -9.9928) -> (108.9626, -22.9936)
  spline S253 degree 3 poles (108.9626, -22.9936) (108.9626, -23.2693) (109.1865, -23.4931) (109.4626, -23.4936) knots 0 0 0 0 1 1 1 1
  line L373 (109.4626, -23.4936) -> (113.4626, -23.4941)
  line L374 (113.4626, -23.4941) -> (113.4626, -23.9937)
  spline S254 degree 3 poles (113.4626, -23.9937) (113.4626, -24.2693) (113.6865, -24.4931) (113.9626, -24.4937) knots 0 0 0 0 1 1 1 1
  line L375 (113.9626, -24.4937) -> (117.9626, -24.4937)
  spline S255 degree 3 poles (117.9626, -24.4937) (118.2388, -24.4931) (118.4626, -24.2693) (118.4626, -23.9937) knots 0 0 0 0 1 1 1 1
  circle A0 centre (27.6475, -44.3518) radius 1.1
  circle A1 centre (27.6475, -8.65) radius 1.1
  circle A2 centre (27.6475, -85.95) radius 1.1
  circle A3 centre (105.8014, -23.5848) radius 1.1
  circle A4 centre (105.9519, -80.7291) radius 1.1
  circle A5 centre (86.9775, -59.4768) radius 1.1
  circle A6 centre (92.2811, -106.4253) radius 1.1
  circle A7 centre (106.737, -4.0898) radius 1.1
  circle A8 centre (140.6317, -84.1371) radius 1.1
  line L376 (2.1623, -87.3399) -> (52.5628, -102.0002)
  line L377 (52.5628, -102.0002) -> (95.2143, -117.7482)
  line L378 (95.2143, -117.7482) -> (136.241, -137.3269)
  arc A9 (140.9605, -135.6379) -> (136.241, -137.3269) centre (137.7622, -134.1393) cw
  line L379 (140.9605, -135.6379) -> (157.6279, -100.0664)
  arc A10 (157.511, -97.1567) -> (157.6279, -100.0664) centre (154.7637, -98.7243) cw
  line L380 (157.511, -97.1567) -> (149.6607, -83.3982)
  arc A11 (149.6607, -83.3982) -> (148.4091, -78.6926) centre (157.9309, -78.6794) cw
  line L381 (148.4091, -78.6926) -> (148.3776, -56.0764)
  arc A12 (146.8839, -54.5848) -> (148.3776, -56.0764) centre (146.8839, -56.0785) cw
  line L382 (146.8839, -54.5848) -> (127.7559, -54.5848)
  arc A13 (127.7559, -54.5848) -> (125.9975, -52.8264) centre (127.7559, -52.8264) cw
  line L383 (125.9975, -52.8264) -> (125.9975, -2.6464)
  arc A14 (124.5064, -1.1127) -> (125.9975, -2.6464) centre (124.4632, -2.6464) cw
  line L384 (124.5064, -1.1127) -> (86.8308, -0.05)
  line L385 (86.8308, -0.05) -> (68.7069, -0.05)
  line L386 (68.7069, -0.05) -> (2.0445, -7.564)
  arc A15 (0.05, -9.7987) -> (2.0445, -7.564) centre (2.296, -9.7959) cw
  line L387 (0.05, -9.7987) -> (0.1425, -84.6522)
  arc A16 (2.1623, -87.3399) -> (0.1424, -84.6522) centre (2.9451, -84.6487) cw
  point P0 (28.7475, -44.3518)
  point P1 (28.7475, -8.65)
  point P2 (28.7475, -85.95)
  point P3 (106.9014, -23.5848)
  point P4 (107.0519, -80.7291)
  point P5 (88.0775, -59.4768)
  point P6 (93.3811, -106.4253)
  point P7 (107.837, -4.0898)
  point P8 (141.7317, -84.1371)
extrude "Extrude18" add sketch "support" along normal blind 1.5 separate body makes body 2
combine "Combine7" operation add target body 2 tool bodies 1
move_body "Move28" bodies 2 to x (1, 0, 0) y (0, 1, 0) z (0, 0, 1) at (0, 0, 10)
extrude "Extrude19" add sketch "support" along normal blind 1.5 separate body makes body 3
move_body "Move29" bodies 3 to x (1, 0, 0) y (0, 1, 0) z (0, 0, 1) at (0, 0, 1.5)
extrude "Extrude20" add sketch "keyplate" along normal blind 1.5 separate body makes body 4
combine "Combine8" operation add target body 3 tool bodies 4